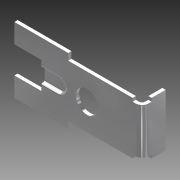
# Autodesk Inventor part: Pusher
Saved by Autodesk Inventor 2011 (Build 150239000, 239)
## iProperties
Shininess: 64.0
Length Units: 11272
Angle Units: 11279
Time Units: 11290
Mass Units: 11286
Length Display Precision: 3
Angle Display Precision: 2
Compacted: True
Part Number: Pusher
Document SubType Name: Sheet Metal
Created: 2002-09-21
Designer: Autodesk, Inc.
Material: Stainless Steel, Austenitic
Project: Inventor Samples
Mass: 2.51018 g
Surface Area: 9.13382 cm^2
Volume: 0.312601 cm^3
Density: 8.03 g/cm^3
Sheet Metal Rule: Default
Density: 0.0
Volumn: 0.0
Area: 0.0
PropertySet Name: Model Information
Control State: 0
Master: False
Checked Out: False
Author: Autodesk, Inc.
Revision Number: A
Autodesk Inventor part; units mm, degrees
ref_plane "YZ Plane" through (0, 0, 0) normal (1, 0, 0) x (0, 1, 0)
ref_plane "XZ Plane" through (0, 0, 0) normal (0, 1, 0) x (-1, 0, 0)
ref_plane "XY Plane" through (0, 0, 0) normal (0, 0, 1) x (1, 0, 0)
sketch "Sketch11" plane through (-15.0876, -6.1976, 0.762) normal (0, 0, 1) x (1, 0, 0)
  line L0 (0, 12.3952) -> (12.7, 12.3952)
  line L1 (12.7, 12.3952) -> (12.7, 13.97)
  line L2 (12.7, 13.97) -> (0, 13.97)
  line L3 (0, 13.97) -> (0, 12.3952)
  line L4 (-6.035, 6.1976) -> (36.2102, 6.1976)
  line L5 (0, 0) -> (12.7, 0)
  line L6 (12.7, 0) -> (12.7, -1.5748)
  line L7 (12.7, -1.5748) -> (0, -1.5748)
  line L8 (0, -1.5748) -> (0, 0)
  dimension "d39" = 1.5748
  dimension "d40" = 12.7
  dimension "d46" = 12.7
  dimension "d47" = 1.5748
  measures "d39" distance of L2.end L0.start
  measures "d40" distance of L1.end L2.end
  measures "d46" distance of L6.end L7.end
  measures "d47" distance of L7.end L5.start
sketch "Sketch9" plane through (-15.0876, -6.1976, 0) normal (0, 0, 1) x (1, 0, 0)
  line L0 (6.35, 4.953) -> (6.35, 7.4422) projected
  line L1 (-6.035, 6.1976) -> (36.2102, 6.1976) projected
  line L2 (6.35, 6.9596) -> (9.525, 6.9596)
  line L3 (9.525, 6.9596) -> (9.525, 5.4356)
  line L4 (9.525, 5.4356) -> (6.35, 5.4356)
  line L5 (6.35, 5.4356) -> (6.35, 6.9596)
  dimension "d34" = 1.524
  dimension "d35" = 3.175
  constraints: 8 end point, 2 parallel, 1 horizontal, 1 perpendicular, 1 point on line, 1 other
  measures "d34" distance of L2.end L3.end
  measures "d35" distance of L2.start L2.end
sketch "Sketch1" plane through (0, 0, 0) normal (0, 0, 1) x (1, 0, 0)
  line L0 (0, 8.6766) -> (0, -8.6766)
  line L1 (-21.1226, 0) -> (21.1226, 0)
  line L2 (-15.0876, 6.1976) -> (15.0876, 6.1976)
  line L3 (15.0876, 6.1976) -> (15.0876, -6.1976)
  line L4 (15.0876, -6.1976) -> (-15.0876, -6.1976)
  line L5 (-15.0876, -6.1976) -> (-15.0876, 6.1976)
  dimension "d0" = 30.1752
  dimension "d1" = 12.3952
  measures "d0" distance of L2.start L2.end
  measures "d1" distance of L4.end L2.start
extrude "Plate1" add sketch "Sketch1" along normal blind 0.762
sketch "Sketch2" plane through (15.0876, -6.1976, 0) normal (-1, 0, 0) x (0, -1, 0)
  line L0 (0, 0) -> (-12.3952, 0)
  line L1 (-12.3952, 0) -> (-12.3952, -4.7752)
  line L2 (-12.3952, -4.7752) -> (0, -4.7752)
  line L3 (0, -4.7752) -> (0, 0)
  constraints: 4 end point, 4 other
sheet face with bend "Flange1" sketch "Sketch2" thickness 0.762 toward (-1, 0, 0) bend radius 0.762 relief straight relief width 0.762 relief depth 0.381
bend "Bend1"
sketch "Sketch3" plane through (-15.0876, -6.1976, 0.762) normal (0, 0, 1) x (1, 0, 0)
  line L0 (30.3748, 12.3952) -> (30.3748, 0) projected
  line L1 (28.6512, 12.3952) -> (30.3748, 12.3952) projected
  line L2 (28.6512, 0) -> (30.3748, 0) projected
  line L3 (28.6512, 0) -> (0, 0) projected
  line L4 (28.6512, 0) -> (28.6512, 12.3952) projected
  line L5 (0, 0) -> (0, 12.3952) projected
  line L6 (0, 12.3952) -> (28.6512, 12.3952) projected
  line L7 (29.513, 0) -> (29.513, 12.3952) projected
  line L8 (30.3748, 12.3952) -> (34.388, 12.3952) projected
  line L9 (34.388, 12.3952) -> (34.388, 0) projected
  line L10 (34.388, 0) -> (30.3748, 0) projected
  line L11 (27.9382, 0) -> (31.0878, 0)
  line L12 (31.0878, 0) -> (31.0878, 0.7874)
  line L13 (31.0878, 0.7874) -> (27.9382, 0.7874)
  line L14 (27.9382, 0.7874) -> (27.9382, 0)
  dimension "d10" = 1.5748
  dimension "d11" = 1.5748
  dimension "d12" = 0.7874
  constraints: 8 end point, 2 parallel, 1 horizontal, 1 perpendicular, 1 point on line
  measures "d10" distance between parallel lines of L14 L7
  measures "d11" distance between parallel lines of L12 L7
  measures "d12" distance of L13.end L11.start
cut across bends "Cut1" sketch "Sketch3" k factor 0.44 contours L13 L12 L10 L0 | L0 L2 L7 L13 | L7 L2 L4 L13 | L4 L3 L14 L13
mirror "Mirror1" about plane through (0, 0, 0) normal (0, 1, 0) of "Cut1"
sketch "Sketch4" plane through (-15.0876, -6.1976, 0.762) normal (0, 0, 1) x (1, 0, 0)
  line L0 (0, 0) -> (0, 12.3952) projected
  line L1 (-6.035, 6.1976) -> (36.2102, 6.1976) projected
  line L2 (0, 9.3726) -> (6.35, 9.3726)
  line L3 (6.35, 9.3726) -> (6.35, 3.0226)
  line L4 (6.35, 3.0226) -> (0, 3.0226)
  line L5 (0, 3.0226) -> (0, 9.3726)
  dimension "d15" = 6.35
  dimension "d16" = 6.35
  constraints: 8 end point, 2 parallel, 1 horizontal, 1 perpendicular, 1 point on line, 1 other
  measures "d15" distance of L2.end L3.end
  measures "d16" distance of L2.start L2.end
extrude "Cut2" cut sketch "Sketch4" against normal blind 0.762
sketch "Sketch5" plane through (-15.0876, -6.1976, 0.762) normal (0, 0, 1) x (1, 0, 0)
  line L0 (-6.035, 6.1976) -> (36.2102, 6.1976) projected
  circle A0 centre (17.1704, 6.1976) radius 2.667
  line L1 (30.1752, 11.6078) -> (30.1752, 0.7874) projected
  dimension "d19" = 5.334
  dimension "d20" = 13.0048
  constraints: 1 centre point, 1 point on line
  measures "d19" diameter of A0
  measures "d20" distance from line of L1 A0.centre
extrude "Cut3" cut sketch "Sketch5" against normal blind 0.762
sketch "Sketch6" plane through (12.8506, -6.1976, 0) normal (0, 0, -1) x (-1, 0, 0)
  line L0 (21.5882, 3.0226) -> (21.5882, 9.3726) projected
  line L1 (-8.272, 6.1976) -> (33.9732, 6.1976) projected
  line L2 (21.5882, 8.5852) -> (17.6258, 8.5852)
  line L3 (17.6258, 3.81) -> (21.5882, 3.81)
  line L4 (21.5882, 3.81) -> (21.5882, 8.5852)
  arc A0 (17.6258, 8.5852) -> (17.6258, 3.81) centre (17.6258, 6.1976) ccw
  dimension "d23" = 4.7752
  dimension "d24" = 3.9624
  constraints: 6 end point, 2 point on circle, 2 point on line, 2 tangent, 1 centre point, 1 horizontal, 1 parallel
  measures "d23" distance of L3.end L2.start
  measures "d24" distance from line of L4 A0.centre
extrude "Extrusion1" add sketch "Sketch6" along normal blind 0.762
sketch "Sketch8" plane through (-15.0876, -6.1976, 0.762) normal (0, 0, 1) x (1, 0, 0)
  line L0 (6.35, 3.81) -> (10.3124, 3.81) projected
  arc A0 (10.3124, 3.81) -> (10.3124, 8.5852) centre (10.3124, 6.1976) ccw projected
  line L1 (10.3124, 8.5852) -> (6.35, 8.5852) projected
  line L2 (6.35, 7.8232) -> (10.3124, 7.8232)
  arc A1 (10.3124, 4.572) -> (10.3124, 7.8232) centre (10.3124, 6.1976) ccw
  line L3 (10.3124, 4.572) -> (6.35, 4.572)
  line L4 (6.35, 7.8232) -> (6.35, 4.572)
  dimension "d29" = 0.762
  constraints: 6 end point, 2 point on circle, 1 centre point, 1 perpendicular, 2 other
  measures "d29" distance between parallel lines of L0 L3
extrude "Extrusion2" cut sketch "Sketch8" against normal blind 0.762
fillet "Fillet3" radius 0.381 6 edges at (-3.1496, 0, 0.762) (-6.7564, -1.6256, 0.762) (-6.7564, 1.6256, 0.762) (-6.7564, -1.6256, 0) (-3.1496, 0, 0) (-6.7564, 1.6256, 0)
fillet "Fillet4" radius 0.381 6 edges at (-6.7564, -2.3876, -0.762) (-2.3876, 0, -0.762) (-6.7564, 2.3876, -0.762) (-6.7564, -2.3876, 0) (-2.3876, 0, 0) (-6.7564, 2.3876, 0)
sheet face with bend "Face2" sketch "Sketch11" thickness 0.762 toward (0, 0, -1) bend radius 0.762 relief straight relief width 0.762 relief depth 0.381
bend "Bend2"
equation "\"d11\" = d10"
equation "\"d12\" = 0.5 * d10"
equation "\"d13\" = Thickness"
equation "\"d17\" = Thickness"
equation "\"d21\" = Thickness"
equation "\"d25\" = Thickness"
equation "\"d29\" = Thickness"
equation "\"d30\" = Thickness"
equation "\"d32\" = 0.5 * Thickness"
equation "\"d33\" = 0.5 * Thickness"
equation "\"d39\" = d47"
equation "\"d46\" = d40"
equation "\"d3\" = BendReliefWidth"
equation "\"d5\" = MinimumRemnant"
equation "\"d9\" = BendRadius"
equation "\"d4\" = BendReliefDepth"
equation "\"d6\" = BendRadius"
equation "\"d41\" = BendRadius"
equation "\"d42\" = BendReliefWidth"
equation "\"d44\" = MinimumRemnant"
equation "\"d43\" = BendReliefDepth"
equation "\"d45\" = BendRadius"
equation "\"BendRadius\" = Thickness"
equation "\"BendReliefWidth\" = Thickness"
equation "\"BendReliefDepth\" = 0.5 * Thickness"
equation "\"CornerReliefSize\" = 4 * Thickness"
equation "\"MinimumRemnant\" = 2 * Thickness"
equation "\"TransitionRadius\" = BendRadius"
equation "\"d2\" = BendRadius"
equation "\"JacobiRadiusSize\" = Thickness"
equation "\"GapSize\" = Thickness"
equation "\"Thickness\" = 0.762"
body "Solid1"
